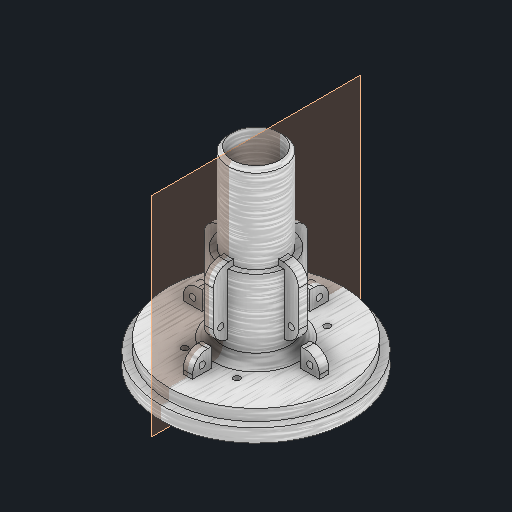
# Autodesk Inventor part: Soporte
Saved by Autodesk Inventor 2025.4 (Build 294407000, 407)
## iProperties
Created: 2024-11-12
Part Number: Soporte
Material: Aluminum 7075
Document SubType Name: Modeling
Designer: j.santaa
Density: 2.81 g/cm^3
Appearance: Satin - Brushed Heavy
Mass: 170.581 g
Surface Area: 426.199 cm^2
Volume: 170.581 cm^3
Author: j.santaa
Autodesk Inventor part; units mm, degrees
ref_plane "XZ Plane" through (0, 0, 0) normal (0, 1, 0) x (-1, 0, 0)
ref_plane "XY Plane" through (0, 0, 0) normal (0, 0, 1) x (1, 0, 0)
sketch "Sketch1" plane through (0, 0, 0) normal (0, 0, 1) x (1, 0, 0)
  circle A0 centre (0, 0) radius 50
  circle A1 centre (0, 0) radius 12.5
  circle A2 centre (0, 0) radius 14.5
  line L0 (-15.5, -15.5) -> (15.5, -15.5) construction
  line L1 (15.5, -15.5) -> (15.5, 15.5) construction
  line L2 (15.5, 15.5) -> (-15.5, 15.5) construction
  line L3 (-15.5, 15.5) -> (-15.5, -15.5) construction
  line L4 (-15.5, -15.5) -> (15.5, 15.5) construction
  line L5 (15.5, -15.5) -> (-15.5, 15.5) construction
  dimension "Diametro" = 100
  dimension "d1" = 25
  dimension "d2" = 2
  dimension "d8" = 31
  constraints: 12 end point, 6 coincident, 3 centre point, 2 midpoint, 2 parallel, 2 perpendicular, 1 horizontal
  measures "Diametro" diameter of A0
  measures "d1" diameter of A1
  measures "d2" radial gap between concentric circles of A1 A2
  measures "d8" distance of L0.end L1.end
extrude "Extrusion1" add sketch "Sketch1" along normal blind 7 contours A0 | A2
extrude "Extrusion2" add sketch "Sketch1" along normal blind 100 contours A2
ref_plane "Work Plane1" through (0, 0, 22) normal (0, 0, 1) x (1, 0, 0)
sketch "Sketch2" plane through (0, 0, 22) normal (0, 0, 1) x (1, 0, 0)
  arc A0 (2.5, 24.8747) -> (-2.5, 24.8747) centre (0, 0) ccw
  line L0 (2.5, 24.8747) -> (2.5, 14.2829)
  line L1 (-2.5, 24.8747) -> (-2.5, 14.2829)
  line L2 (0, -70) -> (0, 70) projected
  circle A1 centre (0, 0) radius 14.5 projected
  point P0 (0, 25)
  dimension "d24" = 5
  dimension "d25" = 25
  dimension "Dedos" = 5
  constraints: 5 point on circle, 4 end point, 1 centre point, 1 coincident, 1 vertical alignment, 1 other
  measures "d24" distance of L1.start L0.start
  measures "d25" distance of point (0, 0) point (0, 25)
  measures "Dedos" distance of L0.end L1.end
extrude "Extrusion3" add sketch "Sketch2" along normal blind 15 contours L0 A1 L2 A0 | L2 A1 L1 A0
sketch "Sketch3" plane through (0, 0, 0) normal (1, 0, 0) x (0, 1, 0)
  line L0 (25, 37) -> (24.8747, 37) projected
  line L1 (14.2829, 22) -> (14.5, 22) projected
  line L2 (25, 22) -> (25, 37) projected
  line L3 (14.2829, 22) -> (14.2829, 37) projected
  circle A0 centre (25.74, 29.5) radius 1.5
  line L4 (0, -7.4) -> (0, 44.4) projected
  point P0 (0, 0)
  point P1 (25, 29.5)
  dimension "d31" = 3
  dimension "d92" = 25.74
  constraints: 1 centre point, 1 coincident, 1 horizontal alignment, 1 midpoint
  measures "d31" diameter of A0
  measures "d92" distance from line of L4 A0.centre
fillet "Fillet2" radius 8 1 edges at (0, 25, 22)
pattern_circular "Circular Pattern1" count 4 over 360 about axis through (0, 0, 0) along (0, 0, 1) of "Fillet2", "Extrusion3"
ref_plane "Plano de trabajo2" through (0, 0, 54) normal (0, 0, 1) x (1, 0, 0)
sketch "Boceto4" plane through (0, 0, 54) normal (0, 0, 1) x (1, 0, 0)
  circle A0 centre (0, 0) radius 17.5
  circle A1 centre (0, 0) radius 14.5 projected
  line L0 (4, -23.75) -> (4, -26.75) projected
  dimension "d54" = 35
  constraints: 1 centre point, 1 coincident
  measures "d54" diameter of A0
extrude "Extrusión5" add sketch "Boceto4" against normal up to surface (47 mm away)
sketch "Boceto5" plane through (0, 0, 37) normal (0, 0, 1) x (0, 1, 0)
  arc A0 (-2.5, -17.3205) -> (2.5, -17.3205) centre (0, 0) ccw projected
  line L0 (-2.5, -17.3205) -> (-2.5, -24.8747) projected
  arc A1 (-2.5, -24.8747) -> (2.5, -24.8747) centre (0, 0) ccw projected
  line L1 (2.5, -24.8747) -> (2.5, -17.3205) projected
  circle A2 centre (0, 0) radius 14.5 projected
  line L2 (2.5, -17.3205) -> (2.5, -14.2829)
  line L3 (-2.5, -17.3205) -> (-2.5, -14.2829)
  constraints: 4 end point, 2 point on circle, 1 parallel, 1 vertical
extrude "Extrusión6" add sketch "Boceto5" along normal blind 20 contours L3 A2 L2 A0 | A0 L1 A1 L0
fillet "Empalme4" radius 8 1 edges at (25, 0, 57)
pattern_circular "Patrón circular2" count 4 over 360 about axis through (0, 0, 54) along (0, 0, -1) of "Extrusión6", "Empalme4"
chamfer "Chaflán1" distance 2 angle 45 1 edges at (-14.5, 0, 100)
sketch "Boceto6" plane through (0, 0, 7) normal (0, 0, 1) x (1, 0, 0)
  circle A0 centre (0, 0) radius 50 projected
  arc A1 (17.3205, 2.5) -> (2.5, 17.3205) centre (0, 0) ccw construction
  line L0 (0, 0) -> (32.476, 18.75) construction
  arc A2 (17.3205, 2.5) -> (2.5, 17.3205) centre (0, 0) ccw construction
  point P0 (16.25, -6.4952)
  point P1 (16.25, 6.4952)
  point P2 (0, 37.5)
  point P3 (-32.476, 18.75)
  point P4 (-32.476, -18.75)
  point P5 (0, -37.5)
  point P6 (32.476, -18.75)
  point P7 (10.8253, 13.75)
  point P8 (15.1554, 8.75)
  dimension "d73" = 360
  dimension "d91" = 37.5
  constraints: 2 end point, 1 point on circle, 1 point on line, 7 other
  measures "d91" distance of L0.start L0.end
sketch "Boceto8" plane through (0, 0, 7) normal (0, 0, 1) x (1, 0, 0)
  circle A0 centre (0, 0) radius 17.5 projected
  circle A1 centre (0, 0) radius 50 projected
  circle A2 centre (0, 0) radius 46
  dimension "Espesor" = 4
  constraints: 1 centre point, 1 coincident
  measures "Espesor" radial gap between concentric circles of A2 A1
extrude "Extrusión8" add sketch "Boceto8" along normal blind 6 contours A2
sketch "Boceto9" plane through (2.5, 14.0104, 54) normal (1, 0, 0) x (0, -1, 0)
  line L0 (16.5104, 0) -> (28.2932, 0) projected
  line L1 (-35.9896, 54) -> (64.0104, 54) projected
  point P0 (1.4018, 24.5)
  point P1 (22.4018, 0)
  dimension "d124" = 21
  dimension "d125" = 29.5
  constraints: 1 midpoint
  measures "d124" horizontal distance of point (22.402, 0) point (1.402, 24.5)
  measures "d125" distance from line of L1 point (1.402, 24.5)
hole "Agujero4" at (2.5, 12.6086, 29.5) direction (-1, 0, 0) diameter 3.4 depth 5 tip angle 118 clearance for "Tornillo de cabeza plana avellanada ISO 2009/7046" size "M3" standard "ISO"
pattern_circular "Patrón circular3" count 4 over 360 about axis through (0, 0, 54) along (0, 0, -1) of "Agujero4"
sketch "Boceto13" plane through (0, 0, 13) normal (0, 0, 1) x (1, 0, 0)
  point P0 (0, 0)
sketch "Boceto15" plane through (0, 0, 0) normal (0, 0, -1) x (-1, 0, 0)
  circle A0 centre (0, 0) radius 27.5 construction
  point P0 (27.5, 0)
  point P1 (13.75, 23.8157)
  point P2 (-13.75, 23.8157)
  point P3 (-27.5, 0)
  point P4 (-13.75, -23.8157)
  point P5 (13.75, -23.8157)
  dimension "d134" = 55
  dimension "d137" = 360
  constraints: 2 horizontal alignment, 1 coincident, 9 other
hole "Agujero8" at (-13.75, -23.8157, 0) at (13.75, -23.8157, 0) at (27.5, 0, 0) at (13.75, 23.8157, 0) at (-13.75, 23.8157, 0) at (-27.5, 0, 0) direction (0, 0, 1) diameter 3.4 end through all clearance for "Tornillo de cabeza cilíndrica ranurada ISO 1207" size "M3" standard "ISO"
sketch "Boceto16" plane through (0, 0, 0) normal (0, 0, -1) x (-1, 0, 0)
  circle A0 centre (0, 0) radius 32.465
  dimension "d146" = 64.93
  constraints: 1 centre point, 1 coincident
  measures "d146" diameter of A0
extrude "Extrusión10" cut sketch "Boceto16" against normal blind 8
sketch "Boceto18" plane through (0, 0, 0) normal (0, 0, -1) x (-1, 0, 0)
  point P0 (0, 0)
  point P1 (-41.233, 0)
  point P2 (-29.1561, -29.1561)
  point P3 (0, -41.233)
  point P4 (29.1561, -29.1561)
  point P5 (41.233, 0)
  point P6 (29.1561, 29.1561)
  point P7 (0, 41.233)
  point P8 (-29.1561, 29.1561)
  dimension "d162" = 41.233
  dimension "d165" = 360
  constraints: 1 horizontal alignment, 9 other
  measures "d162" distance of point (0, 0) point (-41.233, 0)
hole "Agujero10" at (41.233, 0, 0) at (29.1561, -29.1561, 0) at (0, -41.233, 0) at (-29.1561, -29.1561, 0) at (-41.233, 0, 0) at (-29.1561, 29.1561, 0) at (0, 41.233, 0) at (29.1561, 29.1561, 0) direction (0, 0, 1) diameter 2.459 depth 10 thread size "M3x0.5" class "6H" standard "ISO Metric profile"
sketch "Sketch19" plane through (14.2829, -2.5, 54) normal (0, -1, 0) x (1, 0, 0)
  circle A0 centre (6.7167, -24.5) radius 1.7
  line L0 (3.0377, 0) -> (3.0377, -31.9844) projected
  line L1 (3.0377, 0) -> (-11.7829, 0) projected
  point P0 (-14.2829, -54)
  dimension "d174" = 3.4
  dimension "d175" = 3.679
  dimension "d176" = 24.5
  constraints: 1 centre point
  measures "d174" diameter of A0
  measures "d175" distance from line of A0.centre L0
  measures "d176" distance from line of A0.centre L1
hole "Hole11" at (20.9995, -2.5, 29.5) direction (0, 1, 0) diameter 3.4 depth 5
pattern_circular "Circular Pattern4" count 4 over 360 about axis through (0, 0, 0) along (0, 0, 1) of "Hole11"
sketch "Sketch21" plane through (0, 0, 13) normal (0, 0, 1) x (1, 0, 0)
  circle A0 centre (-27.5, 0) radius 1.7 projected
  circle A1 centre (-13.75, 23.8157) radius 1.7 projected
  circle A2 centre (13.75, 23.8157) radius 1.7 projected
  circle A3 centre (27.5, 0) radius 1.7 projected
  circle A4 centre (13.75, -23.8157) radius 1.7 projected
  circle A5 centre (-13.75, -23.8157) radius 1.7 projected
  circle A6 centre (0, 0) radius 46 projected
  circle A7 centre (0, 0) radius 17.5 projected
  line L0 (2.5, -24.8747) -> (2.5, -16.8152) projected
  arc A8 (-2.5, -16.8152) -> (2.5, -16.8152) centre (0, 0) ccw projected
  line L1 (-2.5, -16.8152) -> (-2.5, -24.8747) projected
  arc A9 (-2.5, -24.8747) -> (2.5, -24.8747) centre (0, 0) ccw projected
  line L2 (-2.5, -17.3205) -> (-2.5, -14.2829) projected
  line L3 (-2.5, -14.2829) -> (-2.5, -49.9375)
  circle A10 centre (0, 0) radius 50 projected
  line L4 (2.5, -16.8152) -> (2.5, -14.2829) projected
  line L5 (2.5, -14.2829) -> (2.5, -49.9375)
  circle A11 centre (0, 0) radius 36
  circle A12 centre (0, 0) radius 26
  point P0 (2.5, -25.8795)
  point P1 (-2.5, -25.8795)
  point P2 (-2.5, -35.9131)
  point P3 (2.5, -35.9131)
  dimension "d187" = 10
  dimension "d188" = 10
  constraints: 4 end point, 2 centre point, 2 coincident, 2 point on circle, 1 collinear, 1 vertical, 1 other
  measures "d187" radial gap between concentric circles of A6 A11
  measures "d188" radial gap between concentric circles of A11 A12
extrude "Extrusion12" add sketch "Sketch21" along normal blind 10 contours A12 L5 A11 L3
fillet "Fillet9" radius 8 1 edges at (0, -36, 23)
sketch "Sketch22" plane through (2.5, -35.9131, 13) normal (1, 0, 0) x (0, 0, -1)
  line L0 (-10, 8.0249) -> (-10, 10.0336) projected
  line L1 (0, 10.0336) -> (0, 0) projected
  line L2 (0, 10.0336) -> (-10, 10.0336) projected
  circle A0 centre (-4, 5.0336) radius 1.85
  line L3 (0, 0) -> (-2, 0) projected
  point P0 (13, 35.9131)
  dimension "d193" = 3.7
  dimension "d194" = 5
  dimension "d195" = 4
  constraints: 1 centre point, 1 other
  measures "d193" diameter of A0
  measures "d194" distance from line of L2 A0.centre
  measures "d195" distance from line of L1 A0.centre
hole "Hole12" at (2.5, -30.8795, 17) direction (-1, 0, 0) diameter 3.4 depth 5
pattern_circular "Circular Pattern5" count 4 over 360 about axis through (0, 0, 54) along (0, 0, -1) of "Extrusion12", "Fillet9", "Hole12"
fillet "Fillet11" radius 5 1 edges at (-17.5, 0, 13)
sketch "Sketch23" plane through (0, 0, 8) normal (0, 0, -1) x (-1, 0, 0)
  circle A0 centre (-27.5, 0) radius 1.7 projected
  circle A1 centre (-27.5, 0) radius 1.7
  circle A2 centre (27.5, 0) radius 1.7 projected
  circle A3 centre (27.5, 0) radius 1.7
  point P0 (0, 0)
  constraints: 2 centre point, 2 coincident
extrude "Extrusion13" add sketch "Sketch23" against normal up to surface (5 mm away)
equation "\"d24\" = Dedos"
equation "\"d91\" = 0.375 * Diametro"
body "Solid1"
